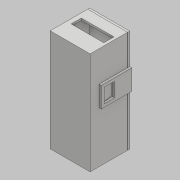
# Autodesk Inventor part: TCampBox
Saved by Autodesk Inventor 2018 (Build 220112000, 112)
## iProperties
Created: 2019-07-02
Part Number: TCampBox
Material: Generic
Document SubType Name: Modeling
Designer: mkivekas
Density: 1 g/cm^3
Appearance: Default
Author: mkivekas
Autodesk Inventor part; units mm, degrees
ref_plane "YZ Plane" through (0, 0, 0) normal (1, 0, 0) x (0, 1, 0)
sketch "Sketch1" plane through (0, 0, 0) normal (0, 1, 0) x (-1, 0, 0)
  line L0 (-9.0266, 15.0024) -> (10.4734, 15.0024)
  line L1 (10.4734, 15.0024) -> (10.4734, -34.9976)
  line L2 (10.4734, -34.9976) -> (-9.0266, -34.9976)
  line L3 (-9.0266, -34.9976) -> (-9.0266, 15.0024)
  point P0 (0, 0)
  dimension "d0" = 19.5
  dimension "d1" = 50
  constraints: 8 end point, 2 parallel, 1 horizontal, 1 perpendicular
  measures "d0" distance of L0.start L0.end
  measures "d1" distance of L0.end L1.end
extrude "Extrusion1" add sketch "Sketch1" along normal blind 1
sketch "Sketch2" plane through (0, 1, 0) normal (0, 1, 0) x (1, 0, 0)
  line L0 (-9.4734, -14.0024) -> (8.0266, -14.0024)
  line L1 (8.0266, -14.0024) -> (8.0266, 33.9976)
  line L2 (8.0266, 33.9976) -> (-9.4734, 33.9976)
  line L3 (-9.4734, 33.9976) -> (-9.4734, -14.0024)
  line L4 (-10.4734, 34.9976) -> (-10.4734, -15.0024) projected
  line L5 (9.0266, -15.0024) -> (9.0266, 34.9976) projected
  line L6 (-10.4734, -15.0024) -> (9.0266, -15.0024) projected
  line L7 (9.0266, 34.9976) -> (-10.4734, 34.9976) projected
  point P0 (0, 0)
  dimension "d4" = 1
  dimension "d5" = 1
  dimension "d6" = 1
  dimension "d7" = 1
  constraints: 8 end point, 2 parallel, 1 horizontal, 1 perpendicular
  measures "d4" distance between parallel lines of L4 L3
  measures "d5" distance between parallel lines of L5 L1
  measures "d6" distance between parallel lines of L6 L0
  measures "d7" distance between parallel lines of L7 L2
extrude "Extrusion2" add sketch "Sketch2" along normal blind 7
sketch "Sketch3" plane through (0, 8, 0) normal (0, 1, 0) x (1, 0, 0)
  line L0 (9.0266, -15.0024) -> (-10.4734, -15.0024) projected
  line L1 (-10.4734, 34.9976) -> (9.0266, 34.9976) projected
  line L2 (-10.4734, -15.0024) -> (9.0266, -15.0024)
  line L3 (9.0266, -15.0024) -> (9.0266, 34.9976)
  line L4 (9.0266, 34.9976) -> (-10.4734, 34.9976)
  line L5 (-10.4734, 34.9976) -> (-10.4734, -15.0024)
  line L6 (-9.4734, 33.9976) -> (-9.4734, -14.0024) projected
  line L7 (8.0266, 33.9976) -> (-9.4734, 33.9976) projected
  line L8 (-9.4734, -14.0024) -> (8.0266, -14.0024)
  line L9 (8.0266, -14.0024) -> (8.0266, 33.9976)
  line L10 (8.0266, 33.9976) -> (-9.4734, 33.9976)
  line L11 (-9.4734, 33.9976) -> (-9.4734, -14.0024)
  line L12 (-9.4734, -14.0024) -> (8.0266, -14.0024) projected
  line L13 (7.7266, -14.0024) -> (-8.2734, -14.0024)
  line L14 (-8.2734, -14.0024) -> (-8.2734, -15.0024)
  line L15 (-8.2734, -15.0024) -> (7.7266, -15.0024)
  line L16 (7.7266, -15.0024) -> (7.7266, -14.0024)
  line L17 (-7.4734, 33.9976) -> (3.2266, 33.9976)
  line L18 (3.2266, 33.9976) -> (3.2266, 34.9976)
  line L19 (3.2266, 34.9976) -> (-7.4734, 34.9976)
  line L20 (-7.4734, 34.9976) -> (-7.4734, 33.9976)
  point P0 (0, 0)
  dimension "d10" = 0.3
  dimension "d11" = 16
  dimension "d12" = 2
  dimension "d13" = 10.7
  constraints: 32 end point, 8 parallel, 4 horizontal, 4 perpendicular, 4 point on line
  measures "d10" distance of L13.start L8.end
  measures "d11" distance between parallel lines of L14 L16
  measures "d12" distance from line of L20 L10.end
  measures "d13" distance from line of L18 L17.start
extrude "Extrusion3" add sketch "Sketch3" along normal blind 10.3 contours L0 L16 L8 L9 L7 L18 L1 L3 | L0 L5 L1 L20 L7 L6 L8 L14
sketch "Sketch4" plane through (0, 18.3, 0) normal (0, 1, 0) x (1, 0, 0)
  line L0 (-10.4734, -15.0024) -> (-10.4734, 34.9976) projected
  line L1 (-10.4734, -15.0024) -> (9.113, -15.0024)
  line L2 (9.113, -15.0024) -> (9.113, 34.9976)
  line L3 (9.113, 34.9976) -> (-10.4734, 34.9976)
  line L4 (-10.4734, 34.9976) -> (-10.4734, -15.0024)
  line L5 (-7.4651, 34.9976) -> (3.2707, 34.9976)
  line L6 (3.2707, 34.9976) -> (3.2707, 27.9976)
  line L7 (3.2707, 27.9976) -> (-7.4651, 27.9976)
  line L8 (-7.4651, 27.9976) -> (-7.4651, 34.9976)
  point P0 (0, 0)
  dimension "d16" = 7
  dimension "d50" = 50
  constraints: 16 end point, 4 parallel, 2 horizontal, 2 perpendicular, 1 point on line
  measures "d16" distance of L7.end L5.start
  measures "d50" distance of L1.end L2.end
sketch "Sketch5" plane through (-8.2734, 8, 15.0024) normal (1, 0, 0) x (0, 0, -1)
  line L0 (1, 0) -> (1, 10.3) projected
  line L1 (0, 0) -> (0, 10.3) projected
  line L2 (1, 10.3) -> (0, 10.3)
  line L3 (0, 10.3) -> (0, 5)
  line L4 (0, 5) -> (1, 5)
  line L5 (1, 5) -> (1, 10.3)
  point P0 (15.0024, -8)
  dimension "d17" = 5
  constraints: 8 end point, 2 parallel, 1 horizontal, 1 perpendicular, 1 point on line
  measures "d17" distance of L1.start L3.end
extrude "Extrusion4" add sketch "Sketch5" along normal blind 17
extrude "Extrusion5" add sketch "Sketch4" along normal blind 1 separate body contours L0 L3 L8 L7 L6 L2 L1
sketch "Sketch6" plane through (9.113, 18.3, 15.0024) normal (1, 0, 0) x (0, 0, -1)
  line L0 (50, 1) -> (0, 1) projected
  line L1 (15, 1) -> (25, 1)
  line L2 (25, 1) -> (25, -14)
  line L3 (25, -14) -> (15, -14)
  line L4 (15, -14) -> (15, 1)
  line L5 (0, 0) -> (0, 1) projected
  point P0 (15.0024, -18.3)
  dimension "d22" = 10
  dimension "d23" = 15
  dimension "d24" = 15
  constraints: 8 end point, 2 parallel, 1 horizontal, 1 perpendicular, 1 point on line
  measures "d22" distance of L2.end L3.end
  measures "d23" distance between parallel lines of L5 L4
  measures "d24" distance of L1.end L2.end
extrude "Extrusion6" add sketch "Sketch6" along normal blind 1 bodies 2
sketch "Sketch7" plane through (-10.4734, 18.3, -34.9976) normal (-1, 0, 0) x (0, 0, 1)
  line L0 (0, 1) -> (50, 1) projected
  line L1 (35, 1) -> (25, 1)
  line L2 (25, 1) -> (25, -14)
  line L3 (25, -14) -> (35, -14)
  line L4 (35, -14) -> (35, 1)
  line L5 (50, 0) -> (50, 1) projected
  point P0 (34.9976, -18.3)
  dimension "d27" = 15
  dimension "d28" = 15
  dimension "d29" = 10
  constraints: 8 end point, 2 parallel, 1 horizontal, 1 perpendicular, 1 point on line
  measures "d27" distance between parallel lines of L5 L4
  measures "d28" distance of L1.end L2.end
  measures "d29" distance of L2.end L3.end
extrude "Extrusion7" add sketch "Sketch7" along normal blind 1 bodies 2
sketch "Sketch8" plane through (-11.4734, 18.3, -34.9976) normal (-1, 0, 0) x (0, 0, 1)
  line L0 (33.5, -12.5) -> (26.5, -12.5)
  line L1 (26.5, -12.5) -> (26.5, -7.5)
  line L2 (26.5, -7.5) -> (33.5, -7.5)
  line L3 (33.5, -7.5) -> (33.5, -12.5)
  line L4 (35, -14) -> (35, 1) projected
  line L5 (25, 1) -> (25, -14) projected
  line L6 (25, -14) -> (35, -14) projected
  point P0 (34.9976, -18.3)
  dimension "d32" = 1.5
  dimension "d33" = 1.5
  dimension "d34" = 5
  dimension "d35" = 1.5
  constraints: 8 end point, 2 parallel, 1 horizontal, 1 perpendicular
  measures "d32" distance between parallel lines of L4 L3
  measures "d33" distance between parallel lines of L5 L1
  measures "d34" distance of L0.end L1.end
  measures "d35" distance between parallel lines of L6 L0
extrude "Extrusion8" cut sketch "Sketch8" against normal blind 25 bodies 2
sketch "Sketch9" plane through (-10.4734, 0, -34.9976) normal (-1, 0, 0) x (0, 0, 1)
  line L0 (33, 6.1) -> (27, 6.1)
  line L1 (27, 6.1) -> (27, 10.5)
  line L2 (27, 10.5) -> (33, 10.5)
  line L3 (33, 10.5) -> (33, 6.1)
  line L4 (33.5, 10.8) -> (33.5, 5.8) projected
  line L5 (26.5, 5.8) -> (26.5, 10.8) projected
  line L6 (33.5, 5.8) -> (26.5, 5.8) projected
  line L7 (26.5, 10.8) -> (33.5, 10.8) projected
  point P0 (34.9976, 0)
  dimension "d38" = 0.5
  dimension "d39" = 0.5
  dimension "d40" = 0.3
  dimension "d41" = 0.3
  constraints: 8 end point, 2 parallel, 1 horizontal, 1 perpendicular
  measures "d38" distance between parallel lines of L4 L3
  measures "d39" distance between parallel lines of L5 L1
  measures "d40" distance between parallel lines of L6 L0
  measures "d41" distance between parallel lines of L7 L2
extrude "Extrusion9" add sketch "Sketch9" along normal blind 0.6 contours L0 L1 L2 L3 bodies 1
ref_plane "Work Plane1" through (-11.0734, 6.1, -7.9976) normal (-0.9908, 0.1351, 0) x (0, 0, 1)
sketch "Sketch10" plane through (-11.0734, 6.1, -7.9976) normal (-0.9908, 0.1351, 0) x (0, 0, 1)
  line L0 (6, 4.4407) -> (6, 0.0811) projected
  line L1 (6, 0.0811) -> (0, 0.0811) projected
  line L2 (6, 4.4407) -> (0, 4.4407)
  line L3 (0, 4.4407) -> (0, 0.0811)
  line L4 (0, 0.0811) -> (6, 0.0811)
  line L5 (6, 0.0811) -> (6, 4.4407)
  point P0 (7.9976, -4.5479)
  constraints: 8 end point, 2 parallel, 1 horizontal, 1 perpendicular
extrude "Extrusion10" cut sketch "Sketch10" along normal blind 0.6 bodies 1
sketch "Sketch11" plane through (9.0266, 0, 15.0024) normal (1, 0, 0) x (0, 0, -1)
  line L0 (17, 6.1) -> (23, 6.1) projected
  line L1 (17, 10.5) -> (17, 6.1) projected
  line L2 (23, 6.1) -> (17, 6.1)
  line L3 (17, 6.1) -> (17, 10.5)
  line L4 (17, 10.5) -> (23, 10.5)
  line L5 (23, 10.5) -> (23, 6.1)
  point P0 (15.0024, 0)
  constraints: 8 end point, 2 parallel, 1 horizontal, 1 perpendicular
extrude "Extrusion11" add sketch "Sketch11" along normal blind 0.6 bodies 1
ref_plane "Work Plane2" through (9.6266, 6.1, -1.9976) normal (0.9908, 0.1351, 0) x (0, 0, -1)
sketch "Sketch12" plane through (9.6266, 6.1, -1.9976) normal (0.9908, 0.1351, 0) x (0, 0, -1)
  line L0 (0, 4.4407) -> (6, 4.4407) projected
  line L1 (6, 0) -> (6, 4.3597) projected
  line L2 (0, 4.4407) -> (6, 4.4407)
  line L3 (6, 4.4407) -> (6, 0)
  line L4 (6, 0) -> (0, 0)
  line L5 (0, 0) -> (0, 4.4407)
  point P0 (-1.9976, -4.7434)
  constraints: 8 end point, 2 parallel, 1 horizontal, 1 perpendicular
extrude "Extrusion12" cut sketch "Sketch12" along normal blind 0.6 bodies 1
body "Solid1"
body "Solid2"
